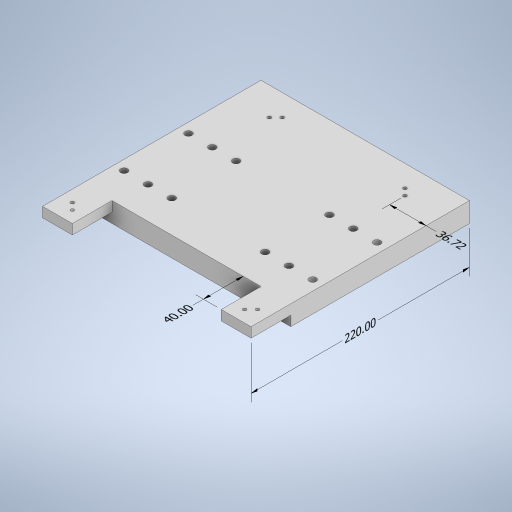
# Autodesk Inventor part: base_back
Saved by Autodesk Inventor 2023 (Build 270158000, 158)
## iProperties
Created: 2022-10-20
Part Number: base_back
Material: Genérico
Document SubType Name: Modeling
Designer: inigo
Density: 1 g/cm^3
Appearance: Valor por defecto
Author: inigo
Autodesk Inventor part; units mm, degrees
ref_plane "YZ Plane" through (0, 0, 0) normal (1, 0, 0) x (0, 1, 0)
ref_plane "XZ Plane" through (0, 0, 0) normal (0, 1, 0) x (-1, 0, 0)
ref_plane "XY Plane" through (0, 0, 0) normal (0, 0, 1) x (1, 0, 0)
sketch "Boceto1" plane through (0, 0, 0) normal (0, 1, 0) x (-1, 0, 0)
  line L0 (105, 90) -> (-105, 90)
  line L1 (-105, 90) -> (-105, -90)
  line L2 (-105, -90) -> (105, -90)
  line L3 (105, -90) -> (105, 90)
  line L4 (105, 90) -> (-105, -90) construction
  line L5 (-105, 90) -> (105, -90) construction
  point P0 (0, 0)
  dimension "d0" = 210
  dimension "d1" = 180
  constraints: 12 end point, 2 midpoint, 2 parallel, 1 horizontal, 1 perpendicular
  measures "d0" distance of L2.end L1.end
  measures "d1" distance of L1.end L0.end
extrude "Extrusión1" add sketch "Boceto1" along normal blind 20
sketch "Boceto2" plane through (0, 20, 0) normal (0, 1, 0) x (1, 0, 0)
  circle A0 centre (-95, -57.83) radius 3.5
  line L0 (-105, -65.43) -> (-37, -65.43)
  line L1 (-37, -65.43) -> (-37, 14.57)
  line L2 (-37, 14.57) -> (-105, 14.57)
  line L3 (-105, 14.57) -> (-105, -65.43)
  line L4 (-71, -65.43) -> (-71, -8.508)
  circle A1 centre (-71, -57.83) radius 3.5
  circle A2 centre (-47, -57.83) radius 3.5
  line L5 (-37, -25.43) -> (-48.2072, -25.43)
  circle A3 centre (-47, 6.97) radius 3.5
  circle A4 centre (-71, 6.97) radius 3.5
  circle A5 centre (-95, 6.97) radius 3.5
  line L6 (0, 0) -> (0, 47.1145)
  circle A6 centre (95, -57.83) radius 3.5
  line L7 (105, -65.43) -> (37, -65.43)
  line L8 (37, -65.43) -> (37, 14.57)
  line L9 (37, 14.57) -> (105, 14.57)
  line L10 (105, 14.57) -> (105, -65.43)
  line L11 (71, -65.43) -> (71, -8.508)
  circle A7 centre (71, -57.83) radius 3.5
  circle A8 centre (47, -57.83) radius 3.5
  line L12 (37, -25.43) -> (48.2072, -25.43)
  circle A9 centre (47, 6.97) radius 3.5
  circle A10 centre (71, 6.97) radius 3.5
  circle A11 centre (95, 6.97) radius 3.5
  circle A12 centre (-65, 65) radius 5
  circle A13 centre (65, 65) radius 5
  circle A14 centre (65, 65) radius 5
  line L13 (0, 0) -> (210, 0)
  line L14 (0, 0) -> (210, 0)
  line L15 (210, 0) -> (105, 0)
  circle A15 centre (40, -25) radius 5
  circle A16 centre (0, -75) radius 10
  line L16 (-105, -90) -> (105, -90) projected
  line L17 (105, 90) -> (-105, 90) projected
  line L18 (-105, 90) -> (-105, -90) projected
  dimension "d4" = 7
  dimension "d5" = 68
  dimension "d6" = 80
  dimension "d7" = 7.6
  dimension "d8" = 10
  dimension "d9" = 7
  dimension "d11" = 24
  dimension "d14" = 10
  dimension "d16" = 10
  dimension "d30" = 20
  dimension "d31" = 0
  dimension "d32" = 15
  dimension "d101" = 25
  dimension "d102" = 40
  constraints: 32 end point, 19 symmetric about line, 17 centre point, 3 horizontal, 3 midpoint, 2 parallel, 2 point on line, 2 vertical, 1 perpendicular, 11 other
  measures "d4" diameter of A0
  measures "d5" distance of L2.end L1.end
  measures "d6" distance of L1.end L0.end
  measures "d7" distance from line of L0 A0.centre
  measures "d8" distance from line of L3 A0.centre
  measures "d9" diameter of A1
  measures "d11" distance of A4.centre A5.centre
  measures "d14" diameter of A12
  measures "d16" diameter of A13
  measures "d30" diameter of A16
  measures "d31" distance from line of L6 A16.centre
  measures "d32" distance from line of L16 A16.centre
  measures "d101" distance from line of L17 A12.centre
  measures "d102" distance from line of L18 A12.centre
extrude "Extrusión2" cut sketch "Boceto2" against normal blind 20 contours A0 | A1 L4 | L4 A1 | A2 | A3 | A4 | A5 | A6 | A7 L11 | L11 A7 | A8 | A9 | A10 | A11
sketch "Boceto7" plane through (-105, 0, 90) normal (0, 0, 1) x (1, 0, 0)
  line L0 (0, 10) -> (29.9999, 10)
  line L1 (29.9999, 20) -> (29.9999, 10)
  line L2 (0, 10) -> (29.9999, 10)
  line L3 (29.9999, 10) -> (29.9999, 20)
  line L4 (29.9999, 20) -> (0, 20)
  line L5 (0, 20) -> (0, 10)
  line L6 (180.0001, 10) -> (210, 10)
  line L7 (210, 10) -> (210, 20)
  line L8 (180.0001, 10) -> (210, 10)
  line L9 (210, 10) -> (210, 20)
  line L10 (210, 20) -> (180.0001, 20)
  line L11 (180.0001, 20) -> (180.0001, 10)
  line L12 (0, 0) -> (0, 20) projected
  line L13 (210, 0) -> (210, 20) projected
  point P0 (105, 0)
  point P1 (0, 10)
  dimension "d79" = 29.9999
  dimension "d80" = 10
  dimension "d81" = 0
  dimension "d82" = 10
  dimension "d83" = 29.9999
  dimension "d84" = 0
  constraints: 24 end point, 4 parallel, 2 horizontal, 2 perpendicular, 1 midpoint
  measures "d79" distance between parallel lines of L1 L5
  measures "d80" distance between parallel lines of L0 L4
  measures "d81" distance from line of point (0, 10) L5
  measures "d82" distance between parallel lines of L10 L6
  measures "d83" distance between parallel lines of L7 L11
  measures "d84" distance between parallel lines of L13 L7
extrude "Extrusión7" add sketch "Boceto7" along normal blind 40
sketch "Boceto8" plane through (0, 20, 0) normal (0, 1, 0) x (1, 0, 0)
  line L0 (-105, -90) -> (-105, -130)
  line L1 (-64.3507, -90) -> (-74.3507, -90)
  line L2 (-105, -130) -> (-75.0001, -130)
  line L3 (-75.0001, -130) -> (-75.0001, -90)
  line L4 (-75.0001, -90) -> (-105, -90)
  line L5 (-55.1959, -89.9497) -> (-75.0001, -90)
  circle A0 centre (-93.25, -111.75) radius 1.75
  circle A1 centre (-86.75, -118.25) radius 1.75
  line L6 (-75.0001, -90) -> (75.0001, -90) projected
  line L7 (0, -90) -> (0, -111.75)
  circle A2 centre (86.75, -118.25) radius 1.75
  circle A3 centre (93.25, -111.75) radius 1.75
  point P0 (0, 0)
  point P1 (-63.4459, -118.25)
  point P2 (-86.75, -111.75)
  point P3 (-105, -16)
  point P4 (86.75, -111.75)
  dimension "d67" = 11.7499
  dimension "d86" = 40
  dimension "d87" = 29.9999
  dimension "d88" = 21.75
  dimension "d89" = 11.75
  dimension "d90" = 28.3003
  dimension "d91" = 11.7499
  constraints: 14 end point, 4 centre point, 3 symmetric about line, 1 midpoint, 1 vertical, 2 other
  measures "d67" distance from line of L3 point (-86.75, -111.75)
  measures "d86" distance between parallel lines of L2 L4
  measures "d87" distance between parallel lines of L0 L3
  measures "d88" vertical distance of L1.start A0.centre
  measures "d89" distance from line of L0 A0.centre
  measures "d90" vertical distance of L5.start A1.centre
  measures "d91" distance from line of L3 A1.centre
hole "Agujero1" at (-86.75, 20, 118.25) at (-93.25, 20, 111.75) at (86.75, 20, 118.25) at (93.25, 20, 111.75) direction (0, -1, 0) diameter 3.5 end through all
sketch "Boceto9" plane through (0, 20, 0) normal (0, 1, 0) x (1, 0, 0)
  circle A0 centre (61.7786, 68.221) radius 1.75
  line L0 (60.0286, 59.971) -> (70.0286, 59.971)
  line L1 (70.0286, 59.971) -> (70.0286, 69.971)
  line L2 (70.0286, 69.971) -> (60.0286, 69.971)
  line L3 (60.0286, 69.971) -> (60.0286, 59.971)
  line L4 (60.0286, 59.971) -> (70.0286, 69.971) construction
  line L5 (70.0286, 59.971) -> (60.0286, 69.971) construction
  circle A1 centre (68.2786, 61.721) radius 1.75
  line L6 (105, 90) -> (-105, 90) projected
  line L7 (-60.0286, 69.971) -> (-60.0286, 59.971)
  line L8 (-70.0286, 59.971) -> (-70.0286, 69.971)
  line L9 (-60.0286, 59.971) -> (-70.0286, 69.971) construction
  line L10 (-70.0286, 59.971) -> (-60.0286, 69.971) construction
  line L11 (-60.0286, 59.971) -> (-70.0286, 59.971)
  circle A2 centre (-68.2786, 61.721) radius 1.75
  line L12 (-70.0286, 69.971) -> (-60.0286, 69.971)
  circle A3 centre (-61.7786, 68.221) radius 1.75
  point P0 (0, 0)
  point P1 (70.0286, 64.971)
  point P2 (-70.0286, 64.971)
  constraints: 24 end point, 4 centre point
extrude "Extrusión8" cut sketch "Boceto9" against normal blind 20 contours A0 | A1 | A3 | A2
